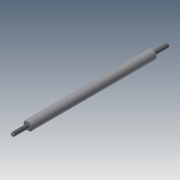
# Autodesk Inventor part: hridel1
Saved by Autodesk Inventor 2013 (Build 170138000, 138)
## iProperties
Created: 2013-05-30
Part Number: hridel1
Material: Generic
Document SubType Name: Modeling
Designer: idle-rug
Density: 1 g/cm^3
Author: idle-rug
Autodesk Inventor part; units mm, degrees
ref_plane "YZ Plane" through (0, 0, 0) normal (1, 0, 0) x (0, 1, 0)
ref_plane "XZ Plane" through (0, 0, 0) normal (0, 1, 0) x (-1, 0, 0)
ref_plane "XY Plane" through (0, 0, 0) normal (0, 0, 1) x (1, 0, 0)
sketch "Sketch1" plane through (0, 0, 0) normal (0, 1, 0) x (-1, 0, 0)
  circle A0 centre (0, 0) radius 3
  dimension "d0" = 6
  constraints: 1 centre point, 1 coincident
  measures "d0" diameter of A0
extrude "Extrusion1" add sketch "Sketch1" along normal blind 82.6
sketch "Sketch2" plane through (0, 82.6, 0) normal (0, 1, 0) x (1, 0, 0)
  circle A0 centre (0, 0) radius 3 projected
hole "Hole1" at (0, 82.6, 0) direction (0, -1, 0) diameter 2.459 depth 8 thread size "M3x0.5" class "6H" standard "ISO Metric profile"
sketch "Sketch3" plane through (0, 0, 0) normal (0, -1, 0) x (1, 0, 0)
  circle A0 centre (0, 0) radius 3 projected
hole "Hole2" at (0, 0, 0) direction (0, 1, 0) diameter 2.459 depth 8 thread size "M3x0.5" class "6H" standard "ISO Metric profile"
chamfer "Chamfer1" distance 0.5 angle 45 2 edges at (3, 0, 0) (3, 82.6, 0)
sketch "Sketch4" plane through (0, 0, 0) normal (0, -1, 0) x (1, 0, 0)
  circle A0 centre (0, 0) radius 1.2295 projected
extrude "Extrusion2" add sketch "Sketch4" along normal blind 10
sketch "Sketch5" plane through (0, 82.6, 0) normal (0, 1, 0) x (1, 0, 0)
  circle A0 centre (0, 0) radius 1.2295 projected
extrude "Extrusion3" add sketch "Sketch5" along normal blind 10
thread "Thread1" size "M3x0.5" class "6g" standard "ANSI Metric M Profile" full length
thread "Thread2" size "M3x0.5" class "6g" standard "ANSI Metric M Profile" full length
chamfer "Chamfer2" distance 0.3 angle 45 1 edges at (-1.2295, -10, 0)
chamfer "Chamfer3" distance 0.3 angle 45 1 edges at (-1.2295, 92.6, 0)
body "Solid1"
